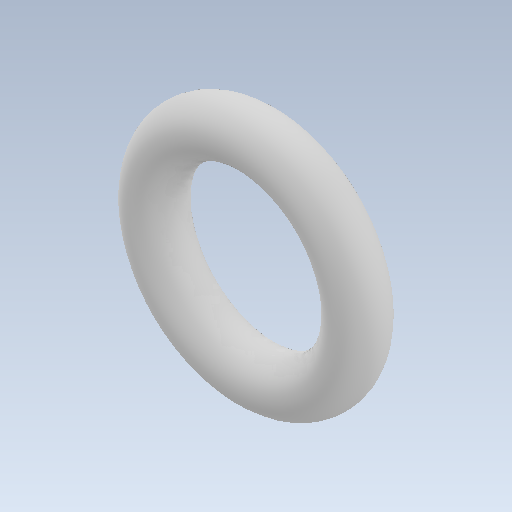
# Autodesk Inventor part: RS 527-9778 Si-O-Ring 5-28ID 1-79 THK 11-32INCH OD
Saved by Autodesk Inventor 2021 (Build 250183000, 183)
## iProperties
Created: 2020-04-22
Part Number: RS 527-9778 Si-O-Ring 5-28ID 1-79 THK 11-32INCH OD
Material: Generic
Document SubType Name: Modeling
Designer: jgray
Density: 1 g/cm^3
Appearance: Default
Author: jgray
Autodesk Inventor part; units mm, degrees
ref_plane "YZ Plane" through (0, 0, 0) normal (1, 0, 0) x (0, 1, 0)
ref_plane "XZ Plane" through (0, 0, 0) normal (0, 1, 0) x (-1, 0, 0)
ref_plane "XY Plane" through (0, 0, 0) normal (0, 0, 1) x (1, 0, 0)
sketch "Sketch1" plane through (0, 0, 0) normal (0, 1, 0) x (-1, 0, 0)
  circle A0 centre (0, 0) radius 3.53 construction
  circle A1 centre (3.53, 0) radius 0.89
  line L0 (0, 5.0651) -> (0, -6.5466) construction
  line L1 (5.5656, 0) -> (-4.0445, 0) construction
  dimension "d0" = 7.06
  dimension "d1" = 1.78
  constraints: 4 end point, 3 point on line, 1 centre point, 1 coincident, 1 horizontal, 1 horizontal alignment, 1 vertical, 2 other
  measures "d1" diameter of A1
revolve "Revolution1" add sketch "Sketch1" angle 360 about axis through (0, 0, 5.0651) along (0, 0, -1)
body "Solid1"
